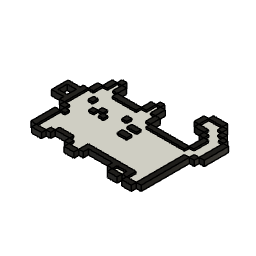
cat (Autodesk Fusion 360 design; units mm, degrees)
Autodesk Fusion 360 part; units mm, degrees
sketch "pisica" plane through (0, 0, 0) normal (0, 0, 1) x (1, 0, 0)
  line L0 (9.5497, 22.6527) -> (9.5497, 36)
  line L1 (9.5497, 36) -> (6.7748, 36)
  line L2 (9.5497, 22.6527) -> (9.5497, 20)
  line L3 (9.5497, 20) -> (12.5, 20)
  line L4 (12.5, 20) -> (12.5, 22.6527)
  line L5 (12.5, 22.6527) -> (9.5497, 22.6527)
  line L6 (12.5, 20) -> (12.5, 17.5)
  line L7 (12.5, 17.5) -> (15, 17.5)
  line L8 (15, 17.5) -> (15, 20)
  line L9 (15, 20) -> (12.5, 20)
  line L10 (12.5, 17.5) -> (9.5, 17.5)
  line L11 (9.5, 17.5) -> (9.5, 4)
  line L12 (9.5, 4) -> (12.5, 4)
  line L13 (12.5, 4) -> (12.5, 17.5)
  line L14 (12.5, 4) -> (12.5, 1.4094)
  line L15 (12.5, 1.4094) -> (18, 1.4094)
  line L16 (18, 1.4094) -> (18, 4)
  line L17 (18, 4) -> (12.5, 4)
  line L18 (18, 4) -> (18, 6.5922)
  line L19 (18, 6.5922) -> (20.4773, 6.5922)
  line L20 (20.4773, 6.5922) -> (20.4773, 4)
  line L21 (20.4773, 4) -> (18, 4)
  line L22 (20.4773, 6.5922) -> (20.4773, 9)
  line L23 (20.4773, 9) -> (28.5, 9)
  line L24 (28.5, 9) -> (28.5, 6.5922)
  line L25 (28.5, 6.5922) -> (20.4773, 6.5922)
  line L26 (28.5, 6.5922) -> (28.5, 3.7713)
  line L27 (28.5, 3.7713) -> (31, 3.7713)
  line L28 (31, 3.7713) -> (31, 6.5922)
  line L29 (31, 6.5922) -> (28.5, 6.5922)
  line L30 (31, 3.7713) -> (31, 1)
  line L31 (31, 1) -> (36.5223, 1)
  line L32 (36.5223, 1) -> (36.5223, 3.7713)
  line L33 (36.5223, 3.7713) -> (31, 3.7713)
  line L34 (36.5223, 3.7713) -> (39, 3.7713)
  line L35 (39, 3.7713) -> (39, 6.6652)
  line L36 (39, 6.6652) -> (52.4582, 6.6652)
  line L37 (52.4582, 6.6652) -> (52.4582, 3.7713)
  line L38 (52.4582, 3.7713) -> (55.2548, 3.7713)
  line L39 (55.2548, 3.7713) -> (55.2548, 1)
  line L40 (55.2548, 1) -> (60.6754, 1)
  line L41 (60.6754, 1) -> (60.6754, 3.7713)
  line L42 (60.6754, 3.7713) -> (63.3199, 3.7713)
  line L43 (63.3199, 3.7713) -> (63.3199, 9)
  line L44 (63.3199, 9) -> (36.5223, 9)
  line L45 (36.5223, 9) -> (36.5223, 3.7713)
  line L46 (55.2548, 3.7713) -> (60.6754, 3.7713)
  line L47 (60.6754, 6.4743) -> (55.2548, 6.4743)
  line L48 (55.2548, 6.4743) -> (55.2548, 3.7713)
  line L49 (60.6754, 6.4743) -> (60.6754, 3.7713)
  line L50 (63.3199, 3.7713) -> (63.3199, 1)
  line L51 (63.3199, 1) -> (68.6426, 1)
  line L52 (68.6426, 1) -> (68.6426, 3.7713)
  line L53 (68.6426, 3.7713) -> (63.3199, 3.7713)
  line L54 (68.6426, 3.7713) -> (71.3968, 3.7713)
  line L55 (71.3968, 3.7713) -> (71.3968, 30.6907)
  line L56 (71.3968, 30.6907) -> (68.6426, 30.6907)
  line L57 (68.6426, 30.6907) -> (68.6426, 3.7713)
  line L58 (71.3968, 30.6907) -> (71.3968, 33.4528)
  line L59 (71.3968, 33.4528) -> (74.1441, 33.4528)
  line L60 (74.1441, 33.4528) -> (74.1441, 30.6907)
  line L61 (74.1441, 30.6907) -> (71.3968, 30.6907)
  line L62 (74.1441, 33.4528) -> (77, 33.4528)
  line L63 (77, 33.4528) -> (77, 47)
  line L64 (77, 47) -> (74.1441, 47)
  line L65 (74.1441, 47) -> (74.1441, 33.4528)
  line L66 (74.1441, 47) -> (71.3684, 47)
  line L67 (71.3684, 47) -> (71.3684, 49.4727)
  line L68 (71.3684, 49.4727) -> (74.1441, 49.4727)
  line L69 (74.1441, 49.4727) -> (74.1441, 47)
  line L70 (71.3684, 49.4727) -> (68.5, 49.4727)
  line L71 (68.5, 49.4727) -> (68.5, 52)
  line L72 (68.5, 52) -> (71.3684, 52)
  line L73 (71.3684, 52) -> (71.3684, 49.4727)
  line L74 (68.5, 52) -> (65.9, 52)
  line L75 (65.9, 52) -> (65.9, 54.9)
  line L76 (65.9, 54.9) -> (68.5, 54.9)
  line L77 (68.5, 54.9) -> (68.5, 52)
  line L78 (65.9, 54.9) -> (58, 54.9)
  line L79 (58, 54.9) -> (58, 57.5763)
  line L80 (58, 57.5763) -> (65.9, 57.5763)
  line L81 (65.9, 57.5763) -> (65.9, 54.9)
  line L82 (58, 54.9) -> (55.3475, 54.9)
  line L83 (55.3475, 54.9) -> (55.3475, 49.4393)
  line L84 (55.3475, 49.4393) -> (58, 49.4393)
  line L85 (58, 49.4393) -> (58, 54.9)
  line L86 (58, 49.4393) -> (58, 47)
  line L87 (58, 47) -> (63.3483, 47)
  line L88 (63.3483, 47) -> (63.3483, 49.4393)
  line L89 (63.3483, 49.4393) -> (58, 49.4393)
  line L90 (63.3483, 47) -> (63.3483, 44.2318)
  line L91 (63.3483, 44.2318) -> (66, 44.2318)
  line L92 (66, 44.2318) -> (66, 47)
  line L93 (66, 47) -> (63.3483, 47)
  line L94 (66, 44.2318) -> (68.6102, 44.2318)
  line L95 (68.6102, 44.2318) -> (68.6102, 36)
  line L96 (68.6102, 36) -> (66, 36)
  line L97 (66, 36) -> (66, 44.2318)
  line L98 (66, 36) -> (44.469, 36)
  line L99 (44.469, 36) -> (44.469, 33.4201)
  line L100 (44.469, 33.4201) -> (66, 33.4201)
  line L101 (66, 33.4201) -> (66, 36)
  line L102 (44.469, 36) -> (41.6973, 36)
  line L103 (41.6973, 36) -> (41.6973, 41.3736)
  line L104 (41.6973, 41.3736) -> (44.469, 41.3736)
  line L105 (44.469, 41.3736) -> (44.469, 36)
  line L106 (41.6973, 41.3736) -> (39, 41.3736)
  line L107 (39, 41.3736) -> (39, 47)
  line L108 (39, 47) -> (41.6973, 47)
  line L109 (41.6973, 47) -> (41.6973, 41.3736)
  line L110 (39, 47) -> (36.5155, 47)
  line L111 (36.5155, 47) -> (36.5155, 49.4074)
  line L112 (36.5155, 49.4074) -> (39, 49.4074)
  line L113 (39, 49.4074) -> (39, 47)
  line L114 (36.5155, 47) -> (33.7824, 47)
  line L115 (33.7824, 47) -> (33.7824, 41.5)
  line L116 (33.7824, 41.5) -> (36.5155, 41.5)
  line L117 (36.5155, 41.5) -> (36.5155, 47)
  line L118 (33.7824, 41.5) -> (20.2941, 41.5)
  line L119 (20.2941, 41.5) -> (20.2941, 38.6364)
  line L120 (20.2941, 38.6364) -> (33.7824, 38.6364)
  line L121 (33.7824, 38.6364) -> (33.7824, 41.5)
  line L122 (20.2941, 41.5) -> (17.6851, 41.5)
  line L123 (17.6851, 41.5) -> (17.6851, 46.6947)
  line L124 (17.6851, 46.6947) -> (20.2941, 46.6947)
  line L125 (20.2941, 46.6947) -> (20.2941, 41.5)
  line L126 (17.6851, 46.6947) -> (15, 46.6947)
  line L127 (15, 46.6947) -> (15, 49.4899)
  line L128 (15, 49.4899) -> (17.6851, 49.4899)
  line L129 (17.6851, 49.4899) -> (17.6851, 46.6947)
  line L130 (15, 46.6947) -> (12.3253, 46.6947)
  line L131 (12.3253, 46.6947) -> (12.3253, 41.2791)
  line L132 (12.3253, 41.2791) -> (15, 41.2791)
  line L133 (15, 41.2791) -> (15, 46.6947)
  line L134 (12.3253, 41.2791) -> (9.6767, 41.2791)
  line L135 (9.6767, 41.2791) -> (9.5497, 36)
  line L136 (12.3915, 36) -> (12.3253, 41.2791)
  line L137 (12.3915, 36) -> (9.5497, 36)
  line L138 (15, 33.5) -> (15, 30.5)
  line L139 (15, 30.5) -> (17.5, 30.5)
  line L140 (17.5, 30.5) -> (17.5, 33.5)
  line L141 (17.5, 33.5) -> (15, 33.5)
  line L142 (33.7804, 33.5) -> (33.7804, 30.5)
  line L143 (33.7804, 30.5) -> (36.5, 30.5)
  line L144 (36.5, 30.5) -> (36.5, 33.5)
  line L145 (36.5, 33.5) -> (33.7804, 33.5)
  line L146 (39.2404, 30.6506) -> (39.2404, 28)
  line L147 (39.2404, 28) -> (44.5, 28)
  line L148 (44.5, 28) -> (44.5, 30.6506)
  line L149 (44.5, 30.6506) -> (39.2404, 30.6506)
  line L150 (39.2404, 25.449) -> (39.2404, 22.5)
  line L151 (39.2404, 22.5) -> (44.5, 22.5)
  line L152 (44.5, 22.5) -> (44.5, 25.449)
  line L153 (44.5, 25.449) -> (39.2404, 25.449)
  line L154 (23, 30.5777) -> (23, 28)
  line L155 (23, 28) -> (25.7862, 28)
  line L156 (25.7862, 28) -> (25.7862, 30.5777)
  line L157 (23, 30.5777) -> (25.7862, 30.5777)
  line L158 (23, 28) -> (20.2563, 28)
  line L159 (20.2563, 28) -> (20.2563, 25.5)
  line L160 (20.2563, 25.5) -> (23, 25.5)
  line L161 (23, 25.5) -> (23, 28)
  line L162 (25.7862, 28) -> (25.7862, 25.5)
  line L163 (25.7862, 25.5) -> (28.5, 25.5)
  line L164 (28.5, 25.5) -> (28.5, 28)
  line L165 (28.5, 28) -> (25.7862, 28)
  line L166 (33.7824, 51) -> (33.7824, 47)
  line L167 (6.7748, 36) -> (6.7748, 22.6527)
  line L168 (6.7748, 22.6527) -> (9.5497, 22.6527)
  line L169 (6.7748, 20) -> (6.7748, 22.6527) construction
  line L170 (6.7748, 32.0418) -> (1.7748, 32.0418)
  line L171 (1.7748, 32.0418) -> (1.7748, 27.0418)
  line L172 (1.7748, 27.0418) -> (6.7748, 27.0418)
  line L173 (6.7748, 34.2728) -> (0, 34.2728)
  line L174 (0, 34.2728) -> (0, 25)
  line L175 (0, 25) -> (6.7748, 25)
  constraint perpendicular L2 L3
  constraint perpendicular L3 L4
  constraint perpendicular L2 L5
  constraint perpendicular L3 L6
  constraint perpendicular L6 L7
  constraint perpendicular L7 L8
  constraint perpendicular L6 L9
  constraint perpendicular L6 L10
  constraint perpendicular L10 L11
  constraint perpendicular L6 L12
  constraint perpendicular L10 L13
  constraint perpendicular L12 L14
  constraint perpendicular L14 L15
  constraint perpendicular L15 L16
  constraint perpendicular L14 L17
  constraint perpendicular L17 L18
  constraint perpendicular L18 L19
  constraint perpendicular L17 L20
  constraint perpendicular L16 L21
  constraint perpendicular L19 L22
  constraint perpendicular L20 L23
  constraint perpendicular L23 L24
  constraint perpendicular L22 L25
  constraint perpendicular L25 L26
  constraint perpendicular L26 L27
  constraint perpendicular L25 L28
  constraint perpendicular L26 L29
  constraint perpendicular L27 L30
  constraint perpendicular L30 L31
  constraint perpendicular L31 L32
  constraint perpendicular L30 L33
  constraint perpendicular L32 L34
  constraint perpendicular L33 L35
  constraint perpendicular L35 L36
  constraint perpendicular L36 L37
  constraint perpendicular L37 L38
  constraint perpendicular L38 L39
  constraint perpendicular L39 L40
  constraint perpendicular L40 L41
  constraint perpendicular L41 L42
  constraint perpendicular L42 L43
  constraint perpendicular L41 L44
  constraint perpendicular L44 L45
  constraint perpendicular L41 L46
  constraint perpendicular L41 L47
  constraint perpendicular L38 L48
  constraint perpendicular L46 L49
  constraint perpendicular L42 L50
  constraint perpendicular L43 L51
  constraint perpendicular L42 L52
  constraint perpendicular L43 L53
  constraint perpendicular L52 L54
  constraint perpendicular L54 L55
  constraint perpendicular L55 L56
  constraint perpendicular L53 L57
  constraint perpendicular L56 L58
  constraint perpendicular L58 L59
  constraint perpendicular L56 L60
  constraint perpendicular L55 L61
  constraint perpendicular L60 L62
  constraint perpendicular L62 L63
  constraint perpendicular L63 L64
  constraint perpendicular L62 L65
  constraint perpendicular L65 L66
  constraint perpendicular L64 L67
  constraint perpendicular L67 L68
  constraint perpendicular L66 L69
  constraint perpendicular L67 L70
  constraint perpendicular L70 L71
  constraint perpendicular L71 L72
  constraint perpendicular L70 L73
  constraint perpendicular L71 L74
  constraint perpendicular L74 L75
  constraint perpendicular L71 L76
  constraint perpendicular L74 L77
  constraint perpendicular L75 L78
  constraint perpendicular L78 L79
  constraint perpendicular L75 L80
  constraint perpendicular L76 L81
  constraint perpendicular L79 L82
  constraint perpendicular L82 L83
  constraint perpendicular L79 L84
  constraint perpendicular L78 L85
  constraint perpendicular L84 L86
  constraint perpendicular L85 L87
  constraint perpendicular L87 L88
  constraint perpendicular L86 L89
  constraint perpendicular L87 L90
  constraint perpendicular L90 L91
  constraint perpendicular L91 L92
  constraint perpendicular L88 L93
  constraint perpendicular L92 L94
  constraint perpendicular L91 L95
  constraint perpendicular L95 L96
  constraint perpendicular L94 L97
  constraint perpendicular L97 L98
  constraint perpendicular L98 L99
  constraint perpendicular L99 L100
  constraint perpendicular L96 L101
  constraint perpendicular L97 L102
  constraint perpendicular L96 L103
  constraint perpendicular L103 L104
  constraint perpendicular L102 L105
  constraint perpendicular L103 L106
  constraint perpendicular L106 L107
  constraint perpendicular L107 L108
  constraint perpendicular L104 L109
  constraint perpendicular L107 L110
  constraint perpendicular L110 L111
  constraint perpendicular L111 L112
  constraint perpendicular L110 L113
  constraint perpendicular L111 L114
  constraint perpendicular L110 L115
  constraint perpendicular L111 L116
  constraint perpendicular L114 L117
  constraint perpendicular L115 L118
  constraint perpendicular L118 L119
  constraint perpendicular L119 L120
  constraint perpendicular L116 L121
  constraint perpendicular L119 L122
  constraint perpendicular L122 L123
  constraint perpendicular L123 L124
  constraint perpendicular L118 L125
  constraint perpendicular L123 L126
  constraint perpendicular L126 L127
  constraint perpendicular L127 L128
  constraint perpendicular L124 L129
  constraint perpendicular L127 L130
  constraint perpendicular L130 L131
  constraint perpendicular L131 L132
  constraint perpendicular L130 L133
  constraint perpendicular L131 L134
  constraint perpendicular L0 L137
  constraint vertical L138
  constraint perpendicular L138 L139
  constraint perpendicular L139 L140
  constraint perpendicular L138 L141
  constraint perpendicular L139 L142
  constraint perpendicular L138 L143
  constraint perpendicular L143 L144
  constraint perpendicular L144 L145
  constraint perpendicular L145 L146
  constraint perpendicular L146 L147
  constraint perpendicular L145 L148
  constraint perpendicular L148 L149
  constraint perpendicular L147 L150
  constraint perpendicular L146 L151
  constraint perpendicular L151 L152
  constraint perpendicular L152 L153
  constraint vertical L154
  constraint perpendicular L154 L155
  constraint perpendicular L155 L156
  constraint perpendicular L154 L157
  constraint perpendicular L154 L158
  constraint perpendicular L158 L159
  constraint perpendicular L159 L160
  constraint perpendicular L158 L161
  constraint perpendicular L155 L162
  constraint perpendicular L156 L163
  constraint perpendicular L163 L164
  constraint perpendicular L156 L165
  constraint perpendicular L2 L168
  constraint perpendicular L1 L167
  constraint perpendicular L168 L169
  constraint coincident L167 L170.start
  constraint perpendicular L167 L170
  constraint perpendicular L170 L171
  constraint coincident L167 L172.end
  constraint perpendicular L167 L172
  constraint coincident L167 L173.start
  constraint perpendicular L167 L173
  constraint perpendicular L170 L174
  constraint coincident L167 L175.end
  constraint perpendicular L167 L175
extrude "Extrude1" add sketch "pisica" along normal blind 3 contours L0 L1 L167 L168 | L2 L3 L4 L5 | L134 L135 L136 L137 | L6 L7 L8 L9 | L130 L131 L132 L133 | L10 L11 L12 L13 | L14 L15 L16 L17 | L126 L127 L128 L129 | L18 L19 L20 L21 | L122 L123 L124 L125 | L22 L23 L24 L25 | L118 L119 L120 L121 | L26 L27 L28 L29 | L114 L115 L116 L117 | L30 L31 L32 L33 | L110 L111 L112 L113 | L34 L35 L36 L37 L38 L42 L43 L44 L45 L47 L48 L49 | L106 L107 L108 L109 | L102 L103 L104 L105 | L50 L51 L52 L53 | L39 L40 L41 L46 | L54 L55 L56 L57 | L98 L99 L100 L101 | L94 L95 L96 L97 | L58 L59 L60 L61 | L90 L91 L92 L93 | L62 L63 L64 L65 | L86 L87 L88 L89 | L66 L67 L68 L69 | L82 L83 L84 L85 | L70 L71 L72 L73 | L78 L79 L80 L81 | L74 L75 L76 L77
extrude "Extrude5" add sketch "pisica" along normal blind 2 contours L0 L4 L5 L7 L8 L9 L13 L17 L18 L19 L22 L23 L24 L28 L29 L33 L43 L44 L45 L53 L56 L57 L58 L59 L65 L66 L67 L70 L71 L74 L75 L78 L85 L88 L89 L92 L93 L94 L95 L96 L99 L100 L101 L102 L103 L106 L107 L110 L116 L117 L119 L120 L121 L122 L123 L126 L132 L133 L136 L137 | L46 L47 L48 L49
extrude "Extrude6" add sketch "pisica" along normal blind 3 contours L138 L139 L140 L141 | L142 L143 L144 L145 | L146 L147 L148 L149 | L150 L151 L152 L153 | L154 L155 L156 L157 | L162 L163 L164 L165 | L158 L159 L160 L161
extrude "Extrude7" add sketch "pisica" along normal blind 3 contours L167 L170 L171 L172 L173 L174 L175
named bodies: "Catto"
